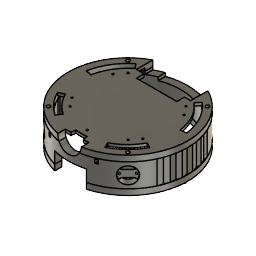
Middle_Layer (Autodesk Fusion 360 design; units mm, degrees)
Autodesk Fusion 360 part; units mm, degrees
note: some values were not read from the file. Set by a fixed rule: which sketch regions a step uses.
sketch "Sketch1" plane through (0, 0, 0) normal (0, 0, 1) x (1, 0, 0)
  circle A0 centre (0, 0) radius 102
  line L0 (0, 0) -> (0, 64) construction
  line L1 (-34.5, 79) -> (34.5, 79)
  line L2 (34.5, 79) -> (34.5, 49)
  line L3 (34.5, 49) -> (-34.5, 49)
  line L4 (-34.5, 49) -> (-34.5, 79)
  line L5 (-34.5, 79) -> (34.5, 49) construction
  line L6 (34.5, 79) -> (-34.5, 49) construction
  point P0 (0, 64)
  dimension "d1" = 204
  dimension "d2" = 64
  dimension "d3" = 69
  dimension "d4" = 30
  constraint coincident A0.centre L0.start
  constraint vertical L0
  constraint horizontal L1
  constraint perpendicular L1 L2
  constraint parallel L1 L3
  constraint parallel L2 L4
  constraint coincident L5 P0
  constraint coincident L6 P0
  constraint coincident P0 L0.end
  measures "d1" diameter of A0
  measures "d2" distance of A0.centre P0
  measures "d3" distance of L2.end L3.end
  measures "d4" distance of L1.end L2.end
extrude "Extrude1" add sketch "Sketch1" along normal blind 5 makes body 1
sketch "Sketch2" plane through (0, 0, 5) normal (0, 0, 1) x (-1, 0, 0)
  line L0 (-34.5, -49) -> (34.5, -49)
  line L1 (34.5, -49) -> (34.5, -79)
  line L2 (34.5, -79) -> (-34.5, -79)
  line L3 (-34.5, -79) -> (-34.5, -49)
  circle A0 centre (0, 0) radius 102
  circle A1 centre (0, 0) radius 70 construction
  line L4 (0, 0) -> (60.6218, 35) construction
  line L5 (0, 0) -> (70, 0) construction
  line L6 (0, 0) -> (60.6218, -35) construction
  line L7 (0, 0) -> (70, 0) construction
  line L8 (0, 0) -> (-60.6218, -35) construction
  line L9 (0, 0) -> (70, 0) construction
  line L10 (0, 0) -> (-60.6218, 35) construction
  line L11 (0, 0) -> (70, 0) construction
  circle A2 centre (60.6218, -35) radius 1.5
  circle A3 centre (60.6218, 35) radius 1.5
  circle A4 centre (-60.6218, -35) radius 1.5
  circle A5 centre (-60.6218, 35) radius 1.5
  dimension "d7" = 140
  dimension "d8" = 30
  dimension "d9" = 30
  dimension "d10" = 150
  dimension "d11" = 150
  dimension "d12" = 3
  dimension "d13" = 3
  dimension "d14" = 3
  dimension "d15" = 3
  constraint concentric A0 A1
  constraint horizontal L5
  constraint coincident A0.centre A1.centre
  constraint horizontal L7
  constraint horizontal L9
  constraint horizontal L11
  constraint coincident L6.end A2.centre
  constraint coincident L4.end A3.centre
  constraint coincident L8.end A4.centre
  constraint coincident L10.end A5.centre
  measures "d7" diameter of A1
  measures "d8" angle of L4 L5
  measures "d9" angle of L6 L7
  measures "d10" angle of L8 L9
  measures "d11" angle of L10 L11
  measures "d12" diameter of A2
  measures "d13" diameter of A3
  measures "d14" diameter of A4
  measures "d15" diameter of A5
extrude "Extrude2" cut sketch "Sketch2" against normal blind 9 contours A2 | A3 | A4 | A5 bodies 1
sketch "Sketch3" plane through (0, 0, 0) normal (0, 0, -1) x (1, 0, 0)
  circle A0 centre (60.6218, 35) radius 1.5
  circle A1 centre (-60.6218, 35) radius 1.5
  circle A2 centre (60.6218, -35) radius 1.5
  circle A3 centre (-60.6218, -35) radius 1.5
  line L0 (-34.5, -49) -> (34.5, -49)
  line L1 (34.5, -49) -> (34.5, -79)
  line L2 (34.5, -79) -> (-34.5, -79)
  line L3 (-34.5, -79) -> (-34.5, -49)
  circle A4 centre (0, 0) radius 102
  circle A5 centre (0, 0) radius 102
  circle A6 centre (0, 0) radius 90
  dimension "d18" = 204
  dimension "d19" = 180
  constraint coincident A4.centre A5.centre
  constraint concentric A5 A6
  measures "d18" diameter of A5
  measures "d19" diameter of A6
extrude "Extrude3" add sketch "Sketch3" along normal blind 5 contours A4 A5 bodies 1
sketch "Sketch4" plane through (0, 0, 0) normal (0, 0, -1) x (1, 0, 0)
  circle A0 centre (0, 0) radius 90
  circle A1 centre (60.6218, 35) radius 1.5
  circle A2 centre (-60.6218, 35) radius 1.5
  circle A3 centre (60.6218, -35) radius 1.5
  circle A4 centre (-60.6218, -35) radius 1.5
  line L0 (-34.5, -49) -> (34.5, -49)
  line L1 (34.5, -49) -> (34.5, -79)
  line L2 (34.5, -79) -> (-34.5, -79)
  line L3 (-34.5, -79) -> (-34.5, -49)
  line L4 (0, 0) -> (0, -49) construction
  line L5 (34.5, -49) -> (-34.5, -49)
  line L6 (-34.5, -49) -> (-34.5, -46.5)
  line L7 (-34.5, -46.5) -> (34.5, -46.5)
  line L8 (34.5, -46.5) -> (34.5, -49)
  dimension "d22" = 2.5
  constraint coincident A0.centre L4.start
  constraint midpoint L0 L4.end
  constraint horizontal L5
  constraint vertical L6
  constraint horizontal L7
  constraint vertical L8
  constraint coincident L0.end L1.start
  measures "d22" distance of L0.end L7.end
extrude "Extrude4" add sketch "Sketch4" along normal blind 54 contours L0 L5 L6 L7 L8 bodies 1
sketch "Sketch5" plane through (0, 0, -5) normal (0, 0, -1) x (1, 0, 0)
  circle A0 centre (0, 0) radius 90
  circle A1 centre (0, 0) radius 102
  circle A2 centre (0, 0) radius 90
  line L0 (0, 0) -> (-88.3346, -51) construction
  line L1 (0, 0) -> (102, 0) construction
  line L2 (0, 0) -> (-88.3346, 51) construction
  line L3 (0, 0) -> (102, 0) construction
  line L4 (0, 0) -> (88.3346, 51) construction
  line L5 (0, 0) -> (102, 0) construction
  line L6 (0, 0) -> (88.3346, -51) construction
  line L7 (0, 0) -> (102, 0) construction
  line L8 (0.3029, -113.7288) -> (0.3029, 125) construction
  line L9 (0, 0) -> (-92.4434, -43.1071) construction
  line L10 (0, 0) -> (102, 0) construction
  line L11 (125, 0) -> (-125, 0) construction
  line L12 (0, 0) -> (-95.8486, -34.8861) construction
  line L13 (0, 0) -> (102, 0) construction
  line L14 (0, 0) -> (-98.5244, -26.3995) construction
  line L15 (0, 0) -> (102, 0) construction
  line L16 (0, 0) -> (-100.4504, -17.7121) construction
  line L17 (0, 0) -> (102, 0) construction
  line L18 (0, 0) -> (-101.6119, -8.8899) construction
  line L19 (0, 0) -> (102, 0) construction
  line L20 (0, 0) -> (-88.3346, 51) construction
  line L21 (0, 0) -> (-92.4434, 43.1071) construction
  line L22 (0, 0) -> (-95.8486, 34.8861) construction
  line L23 (0, 0) -> (-98.5244, 26.3995) construction
  line L24 (0, 0) -> (-100.4504, 17.7121) construction
  line L25 (0, 0) -> (-101.6119, 8.8899) construction
  line L26 (-82.2724, -47.5) -> (-88.3346, -51)
  line L27 (-86.0992, -40.1487) -> (-92.4434, -43.1071)
  line L28 (-82.2724, 47.5) -> (-88.3346, 51)
  line L29 (-86.0992, 40.1487) -> (-92.4434, 43.1071)
  line L30 (-92.4434, -43.1071) -> (-94.909, -34.544)
  line L31 (-94.909, -34.544) -> (-90.6308, -42.2618)
  line L32 (-94.909, -34.544) -> (-96.5926, -25.8819)
  line L33 (-94.909, -34.544) -> (-98.5244, -26.3995)
  line L34 (-96.5926, -25.8819) -> (-99.4656, -17.5385)
  line L35 (-99.4656, -17.5385) -> (-98.5244, -26.3995)
  line L36 (-99.4656, -17.5385) -> (-99.6195, -8.7156)
  line L37 (-99.4656, -17.5385) -> (-101.6119, -8.8899)
  line L38 (-99.6195, -8.7156) -> (-101, 0)
  line L39 (-101, 0) -> (-101.6119, -8.8899)
  line L40 (-101, 0) -> (-99.6195, 8.7156)
  line L41 (-101, 0) -> (-101.6119, 8.8899)
  line L42 (-99.6195, 8.7156) -> (-99.4656, 17.5385)
  line L43 (-99.4656, 17.5385) -> (-101.6119, 8.8899)
  line L44 (-99.4656, 17.5385) -> (-96.5926, 25.8819)
  line L45 (-99.4656, 17.5385) -> (-98.5244, 26.3995)
  line L46 (-96.5926, 25.8819) -> (-94.909, 34.544)
  line L47 (-94.909, 34.544) -> (-98.5244, 26.3995)
  line L48 (-94.909, 34.544) -> (-90.6308, 42.2618)
  line L49 (-94.909, 34.544) -> (-92.4434, 43.1071)
  line L50 (-90.6308, -42.2618) -> (-89.2708, -32.4919)
  line L51 (-89.2708, -32.4919) -> (-96.5926, -25.8819)
  line L52 (-96.5926, -25.8819) -> (-93.5567, -16.4966)
  line L53 (-93.5567, -16.4966) -> (-99.6195, -8.7156)
  line L54 (-99.6195, -8.7156) -> (-95, 0)
  line L55 (-95, 0) -> (-99.6195, 8.7156)
  line L56 (-99.6195, 8.7156) -> (-93.5567, 16.4966)
  line L57 (-93.5567, 16.4966) -> (-96.5926, 25.8819)
  line L58 (-96.5926, 25.8819) -> (-89.2708, 32.4919)
  line L59 (-89.2708, 32.4919) -> (-90.6308, 42.2618)
  line L60 (-91.763, -24.5878) -> (-91.763, 24.5878)
  arc A3 (-82.2724, 47.5) -> (-91.763, 24.5878) centre (0, 0) ccw
  arc A4 (-91.763, -24.5878) -> (-82.2724, -47.5) centre (0, 0) ccw
  line L61 (0.6059, 0) -> (88.9405, -51) construction
  line L62 (0.6059, 0) -> (93.0493, -43.1071) construction
  line L63 (0.6059, 0) -> (96.4545, -34.8861) construction
  line L64 (0.6059, 0) -> (99.1303, -26.3995) construction
  line L65 (0.6059, 0) -> (101.0563, -17.7121) construction
  line L66 (0.6059, 0) -> (102.2178, -8.8899) construction
  line L67 (-124.3941, 0) -> (125.6059, 0) construction
  line L68 (0.6059, 0) -> (102.2178, 8.8899) construction
  line L69 (0.6059, 0) -> (101.0563, 17.7121) construction
  line L70 (0.6059, 0) -> (99.1303, 26.3995) construction
  line L71 (0.6059, 0) -> (96.4545, 34.8861) construction
  line L72 (0.6059, 0) -> (93.0493, 43.1071) construction
  line L73 (0.6059, 0) -> (88.9405, 51) construction
  line L74 (92.5513, -42.8749) -> (86.2071, -39.9165)
  line L75 (88.3346, -51) -> (82.2724, -47.5)
  line L76 (88.3346, 51) -> (82.2724, 47.5)
  line L77 (92.5513, 42.8749) -> (86.2071, 39.9165)
  line L78 (92.5513, -42.8749) -> (94.9796, -34.3492)
  line L79 (94.9796, -34.3492) -> (90.7179, -42.0199)
  line L80 (94.9796, -34.3492) -> (98.5649, -26.248)
  line L81 (94.9796, -34.3492) -> (96.6331, -25.7304)
  line L82 (98.5649, -26.248) -> (99.4838, -17.4348)
  line L83 (99.4838, -17.4348) -> (96.6331, -25.7304)
  line L84 (99.4838, -17.4348) -> (101.6164, -8.8373)
  line L85 (99.4838, -17.4348) -> (99.6241, -8.663)
  line L86 (101.6164, -8.8373) -> (101, 0)
  line L87 (101, 0) -> (99.6241, -8.663)
  line L88 (101, 0) -> (101.6164, 8.8373)
  line L89 (101, 0) -> (99.6241, 8.663)
  line L90 (101.6164, 8.8373) -> (99.4838, 17.4348)
  line L91 (99.4838, 17.4348) -> (99.6241, 8.663)
  line L92 (99.4838, 17.4348) -> (98.5649, 26.248)
  line L93 (99.4838, 17.4348) -> (96.6331, 25.7304)
  line L94 (98.5649, 26.248) -> (94.9796, 34.3492)
  line L95 (96.6331, 25.7304) -> (94.9796, 34.3492)
  line L96 (94.9796, 34.3492) -> (92.5513, 42.8749)
  line L97 (94.9796, 34.3492) -> (90.7387, 42.0296)
  line L98 (90.7387, 42.0296) -> (89.3415, 32.2971)
  line L99 (89.3415, 32.2971) -> (96.6331, 25.7304)
  line L100 (96.6331, 25.7304) -> (93.5749, 16.393)
  line L101 (93.5749, 16.393) -> (99.6241, 8.663)
  line L102 (99.6241, 8.663) -> (95, 0)
  line L103 (95, 0) -> (99.6241, -8.663)
  line L104 (99.6241, -8.663) -> (93.5749, -16.393)
  line L105 (93.5749, -16.393) -> (96.6331, -25.7304)
  line L106 (96.6331, -25.7304) -> (89.3415, -32.2971)
  line L107 (89.3415, -32.2971) -> (90.7179, -42.0199)
  line L108 (89.3415, -32.2971) -> (93.5749, 16.393)
  arc A5 (86.7536, 49.7374) -> (86.6025, 50) centre (0, 0) ccw
  arc A6 (87.4686, -50.5) -> (87.6196, -50.2374) centre (0, 0) ccw
  arc A7 (87.6196, 50.2374) -> (87.4686, 50.5) centre (0, 0) ccw
  arc A8 (-92.4434, -43.1071) -> (92.5513, -42.8749) centre (0, 0) ccw
  arc A9 (92.5513, 42.8749) -> (-92.4434, 43.1071) centre (0, 0) ccw
  arc A10 (82.2724, -47.5) -> (89.3415, -32.2971) centre (0, 0) ccw
  arc A11 (93.5749, 16.393) -> (82.2724, 47.5) centre (0, 0) ccw
  arc A12 (86.6025, -50) -> (86.7536, -49.7374) centre (0, 0) ccw
  arc A13 (90.7387, -42.0296) -> (90.8667, -41.7522) centre (0, 0) ccw
  line L109 (82.2724, -47.5) -> (77.9423, -45)
  line L110 (86.2071, -39.9165) -> (81.6756, -37.8034)
  line L111 (86.2071, 39.9165) -> (81.6756, 37.8034)
  line L112 (82.2724, 47.5) -> (77.9423, 45)
  line L113 (-77.9423, -45) -> (-82.2724, -47.5)
  line L114 (-81.5677, -38.0356) -> (-86.0992, -40.1487)
  line L115 (-77.9423, 45) -> (-82.2724, 47.5)
  line L116 (-81.5677, 38.0356) -> (-86.0992, 40.1487)
  dimension "d25" = 204
  dimension "d26" = 180
  dimension "d27" = 150
  dimension "d28" = 150
  dimension "d29" = 30
  dimension "d30" = 30
  dimension "d31" = 155
  dimension "d32" = 160
  dimension "d33" = 165
  dimension "d34" = 170
  dimension "d35" = 175
  dimension "d36" = 190
  dimension "d37" = 202
  dimension "d38" = 200
  constraint coincident A0.centre A1.centre
  constraint horizontal L1
  constraint horizontal L3
  constraint horizontal L5
  constraint horizontal L7
  constraint vertical L8
  constraint horizontal L10
  constraint horizontal L11
  constraint horizontal L13
  constraint horizontal L15
  constraint horizontal L17
  constraint horizontal L19
  constraint symmetric A0.centre L11 A1.centre
  constraint symmetric L0.end L11 L2.end
  constraint symmetric L9.end L11 L21.end
  constraint symmetric L11 L12.end L22.end
  constraint symmetric L11 L14.end L23.end
  constraint symmetric L11 A0.centre A1.centre
  constraint symmetric L11 L16.end L24.end
  constraint symmetric L11 L18.end L25.end
  constraint coincident L0 L26.start
  constraint coincident L27.start A4
  constraint coincident L9 L27.start
  constraint coincident L20 L28.start
  constraint coincident L21 L29.start
  constraint coincident L29.start A3
  constraint coincident L12 L30.end
  constraint coincident L27 L31.end
  constraint coincident L14 L32.end
  constraint coincident L16 L34.end
  constraint coincident L18 L36.end
  constraint coincident L11 L38.end
  constraint coincident L25 L40.end
  constraint coincident L24 L42.end
  constraint coincident L23 L44.end
  constraint coincident L22 L46.end
  constraint coincident L29 L48.end
  constraint coincident L12 L50.end
  constraint coincident L50.end A4
  constraint coincident L16 L52.end
  constraint coincident L11 L54.end
  constraint coincident L24 L56.end
  constraint coincident L58.end A3
  constraint coincident L22 L58.end
  constraint coincident L14 L60.start
  constraint coincident L23 L60.end
  constraint concentric A3 A11
  constraint coincident L6 L75.end
  constraint coincident L6 A12.start
  constraint coincident L6 A6.start
  constraint coincident L4 L76.end
  constraint coincident L4 A5.end
  constraint coincident L4 A7.end
  constraint concentric A3 A4
  constraint symmetric A0.centre L8 L61.start
  constraint symmetric L0.end L8 L61.end
  constraint symmetric L2.end L8 L73.end
  constraint symmetric L8 A0.centre L61.start
  constraint symmetric L8 L9.end L62.end
  constraint symmetric L8 L11.start L67.start
  constraint symmetric L8 L11.end L67.end
  constraint symmetric L8 L12.end L63.end
  constraint symmetric L8 L14.end L64.end
  constraint symmetric L8 L16.end L65.end
  constraint symmetric L8 L18.end L66.end
  constraint symmetric L8 L21.end L72.end
  constraint symmetric L8 L22.end L71.end
  constraint symmetric L8 L23.end L70.end
  constraint symmetric L8 L24.end L69.end
  constraint symmetric L8 L25.end L68.end
  constraint coincident L62 L74.start
  constraint coincident L62 L74.end
  constraint coincident L74.end A10
  constraint coincident L72 L77.start
  constraint coincident L77.end A11
  constraint coincident L72 L77.end
  constraint coincident L63 L78.end
  constraint coincident L62 L79.end
  constraint coincident L64 L80.end
  constraint coincident A1 L80.end
  constraint coincident L64 L81.end
  constraint coincident L65 L82.end
  constraint coincident L66 L84.end
  constraint coincident L66 L85.end
  constraint coincident L68 L88.end
  constraint coincident L68 L89.end
  constraint coincident L69 L90.end
  constraint coincident L70 L92.end
  constraint coincident L70 L93.end
  constraint coincident L71 L94.end
  constraint coincident L77 L97.end
  constraint coincident L98.end A11
  constraint coincident L71 L98.end
  constraint coincident L69 L100.end
  constraint coincident L65 L104.end
  constraint coincident L63 L106.end
  constraint coincident L73 A5.start
  constraint concentric A5 A13
  constraint coincident L73 A7.start
  constraint concentric A6 A7
  constraint concentric A8 A9
  constraint concentric A10 A11
  constraint coincident L79 A13.end
  constraint coincident L61 A6.end
  constraint coincident L61 A12.end
  constraint coincident L62 A13.start
  constraint concentric A12 A13
  constraint coincident A2 L109.end
  constraint coincident L6 L109.end
  constraint coincident L62 L110.end
  constraint coincident A2 L110.end
  constraint coincident L72 L111.end
  constraint coincident A2 L111.end
  constraint coincident A2 L112.end
  constraint coincident L4 L112.end
  constraint coincident L0 L113.start
  constraint coincident A2 L113.start
  constraint coincident L9 L114.start
  constraint coincident A2 L114.start
  constraint coincident L2 L115.start
  constraint coincident A2 L115.start
  constraint parallel L28 L115
  constraint coincident A2 L116.start
  constraint coincident L21 L116.start
  measures "d25" diameter of A8
  measures "d26" diameter of A2
  measures "d27" angle of L0 L1
  measures "d28" angle of L2 L3
  measures "d29" angle of L4 L5
  measures "d30" angle of L6 L7
  measures "d31" angle of L9 L10
  measures "d32" angle of L12 L13
  measures "d33" angle of L14 L15
  measures "d34" angle of L16 L17
  measures "d35" angle of L18 L19
  measures "d36" diameter of A10
  measures "d37" diameter of A6
  measures "d38" diameter of A12
extrude "Extrude5" add sketch "Sketch5" along normal blind 40 separate body contours A0 A2 A11 L111 L112 | A0 A2 A10 L109 L110 | A0 A1 A2 L28 L76 A9 L112 L115 | A1 L76 L77 A9 A11 | L77 L98 A11 | A0 A1 A2 L26 L75 A8 L109 L113 | L74 L107 A10 | A1 L74 L75 A8 A10 | A0 A2 A3 L115 L116 | L77 L96 L97 | L99 L100 A11 | A0 A2 A4 L113 L114 | L101 L102 L103 L104 L105 L106 L108 | A1 L28 L29 A3 A9 | L92 L93 L94 L95 | A1 L26 L27 A4 A8 | L74 L78 L79 A13 | L80 L81 L82 L83 | L29 L59 A3 | L88 L89 L90 L91 | L27 L50 A4 | L84 L85 L86 L87 | L29 L48 L49 | L51 L52 L53 L54 L55 L56 L57 L58 L60 A3 A4 | L27 L30 L31 | L44 L45 L46 L47 | L32 L33 L34 L35 | L40 L41 L42 L43 | L36 L37 L38 L39 makes body 2 at (-87.956, 51.6502, -18.3333)
sketch "Sketch6" plane through (0, 0, -45) normal (0, 0, -1) x (1, 0, 0)
  line L0 (86.2071, -39.9165) -> (81.6756, -37.8034)
  arc A0 (-81.5677, -38.0356) -> (81.6756, -37.8034) centre (0, 0) ccw
  line L1 (-81.5677, -38.0356) -> (-86.0992, -40.1487)
  arc A1 (-89.2708, -32.4919) -> (-86.0992, -40.1487) centre (0, 0) ccw
  line L2 (-89.2708, -32.4919) -> (-90.6308, -42.2618)
  line L3 (-90.6308, -42.2618) -> (-94.909, -34.544)
  line L4 (-94.909, -34.544) -> (-92.4434, -43.1071)
  arc A2 (-92.4434, -43.1071) -> (92.5513, -42.8749) centre (0, 0) ccw
  line L5 (92.5513, -42.8749) -> (94.9796, -34.3492)
  line L6 (94.9796, -34.3492) -> (90.8667, -41.7522)
  arc A3 (90.7387, -42.0296) -> (90.8667, -41.7522) centre (0, 0) ccw
  line L7 (90.7387, -42.0296) -> (90.7179, -42.0199)
  line L8 (90.7179, -42.0199) -> (89.3415, -32.2971)
  arc A4 (86.2071, -39.9165) -> (89.3415, -32.2971) centre (0, 0) ccw
  circle A5 centre (0, 0) radius 102
  circle A6 centre (0, 0) radius 90
  dimension "d41" = 204
  dimension "d42" = 180
  constraint concentric A3 A5
  constraint concentric A5 A6
  measures "d41" diameter of A5
  measures "d42" diameter of A6
extrude "Extrude6" add sketch "Sketch6" along normal blind 10 separate body contours L0 A0 L1 A1 L2 L3 L4 A2 L5 L6 A3 L7 L8 A4 A5 A6 | L0 L1 A1 L2 L3 L4 L5 L6 A3 L7 L8 A4 A5 A6 makes body 3
sketch "Sketch7" plane through (0, 0, -55) normal (0, 0, -1) x (1, 0, 0)
  circle A0 centre (0, 0) radius 90
  circle A1 centre (0, 0) radius 102
  circle A2 centre (0, 0) radius 96 construction
  circle A3 centre (96, 0) radius 2.975
  circle A4 centre (-96, 0) radius 2.975
  dimension "d45" = 192
  dimension "d46" = 5.95
  dimension "d47" = 5.95
  constraint coincident A0.centre A1.centre
  constraint coincident A2 A3.centre
  constraint coincident A2 A4.centre
  measures "d45" diameter of A2
  measures "d46" diameter of A3
  measures "d47" diameter of A4
extrude "Extrude7" add sketch "Sketch7" along normal blind 3.95 contours A3 | A4 bodies 3
sketch "Sketch8" plane through (0, 0, 0) normal (0, 0, -1) x (1, 0, 0)
  line L0 (-34.5, -49) -> (-34.5, -46.5)
  line L1 (-34.5, -46.5) -> (34.5, -46.5)
  line L2 (34.5, -46.5) -> (34.5, -49)
  line L3 (34.5, -49) -> (34.5, -79)
  line L4 (34.5, -79) -> (-34.5, -79)
  line L5 (-34.5, -79) -> (-34.5, -49)
  circle A0 centre (-60.6218, -35) radius 1.5
  circle A1 centre (60.6218, -35) radius 1.5
  circle A2 centre (-60.6218, 35) radius 1.5
  circle A3 centre (60.6218, 35) radius 1.5
  circle A4 centre (0, 0) radius 90
  circle A5 centre (0, 0) radius 70 construction
  line L6 (0, 0) -> (0, 70) construction
  line L7 (0, 0) -> (49.4975, 49.4975) construction
  line L8 (0, 0) -> (49.4975, -49.4975) construction
  line L9 (0, 0) -> (70, 0) construction
  line L10 (0, 0) -> (-49.4975, -49.4975) construction
  line L11 (0, 0) -> (70, 0) construction
  line L12 (0, 0) -> (-49.4975, 49.4975) construction
  line L13 (0, 0) -> (70, 0) construction
  circle A6 centre (0, 70) radius 1.5
  circle A7 centre (49.4975, 49.4975) radius 1.5
  circle A8 centre (-49.4975, 49.4975) radius 1.5
  circle A9 centre (49.4975, -49.4975) radius 1.5
  circle A10 centre (-49.4975, -49.4975) radius 1.5
  dimension "d50" = 140
  dimension "d51" = 135
  dimension "d52" = 45
  dimension "d53" = 135
  dimension "d54" = 135
  dimension "d55" = 3
  dimension "d56" = 3
  dimension "d57" = 3
  dimension "d58" = 3
  dimension "d59" = 3
  constraint concentric A4 A5
  constraint coincident A4.centre A5.centre
  constraint coincident A5 L6.end
  constraint vertical L6
  constraint horizontal L9
  constraint horizontal L11
  constraint horizontal L13
  constraint coincident L6.end A6.centre
  constraint coincident L7.end A7.centre
  constraint coincident L12.end A8.centre
  constraint coincident L8.end A9.centre
  constraint coincident L10.end A10.centre
  measures "d50" diameter of A5
  measures "d51" angle of L6 L7
  measures "d52" angle of L8 L9
  measures "d53" angle of L10 L11
  measures "d54" angle of L12 L13
  measures "d55" diameter of A6
  measures "d56" diameter of A7
  measures "d57" diameter of A8
  measures "d58" diameter of A9
  measures "d59" diameter of A10
extrude "Extrude8" cut sketch "Sketch8" against normal blind 8 contours A6 | A7 | A8 | A9 | A10 bodies 1
sketch "Sketch9" plane through (0, 0, 0) normal (0, 0, -1) x (1, 0, 0)
  circle A0 centre (49.4975, 49.4975) radius 1.5
  circle A1 centre (-49.4975, -49.4975) radius 1.5
  circle A2 centre (-49.4975, 49.4975) radius 1.5
  circle A3 centre (49.4975, -49.4975) radius 1.5
  circle A4 centre (0, 70) radius 1.5
  line L0 (-34.5, -49) -> (-34.5, -46.5)
  line L1 (-34.5, -46.5) -> (34.5, -46.5)
  line L2 (34.5, -46.5) -> (34.5, -49)
  line L3 (34.5, -49) -> (34.5, -79)
  line L4 (34.5, -79) -> (-34.5, -79)
  line L5 (-34.5, -79) -> (-34.5, -49)
  circle A5 centre (-60.6218, -35) radius 1.5
  circle A6 centre (60.6218, -35) radius 1.5
  circle A7 centre (-60.6218, 35) radius 1.5
  circle A8 centre (60.6218, 35) radius 1.5
  circle A9 centre (0, 0) radius 90
  line L6 (0, 0) -> (0, 55) construction
  line L7 (40.5, 38.5) -> (-40.5, 38.5) construction
  line L8 (-40.5, 38.5) -> (-40.5, 71.5) construction
  line L9 (-40.5, 71.5) -> (40.5, 71.5) construction
  line L10 (40.5, 71.5) -> (40.5, 38.5) construction
  line L11 (40.5, 38.5) -> (-40.5, 71.5) construction
  line L12 (-40.5, 38.5) -> (40.5, 71.5) construction
  circle A10 centre (-40.5, 71.5) radius 2.9
  line L13 (-40.5, 71.5) -> (16.5, 71.5) construction
  line L14 (16.5, 71.5) -> (16.5, 41.5) construction
  circle A11 centre (16.5, 41.5) radius 2.9
  point P0 (0, 55)
  dimension "d62" = 55
  dimension "d63" = 81
  dimension "d64" = 33
  dimension "d65" = 5.8
  dimension "d66" = 57
  dimension "d67" = 30
  dimension "d68" = 5.8
  constraint coincident A9.centre L6.start
  constraint perpendicular L4 L6
  constraint horizontal L7
  constraint perpendicular L7 L8
  constraint parallel L7 L9
  constraint parallel L8 L10
  constraint coincident L11 P0
  constraint coincident L12 P0
  constraint coincident P0 L6.end
  constraint coincident L8.end L9.start
  constraint parallel L9 L13
  constraint perpendicular L13 L14
  constraint coincident L14.end A11.centre
  measures "d62" distance of A9.centre P0
  measures "d63" distance of L8.end L9.end
  measures "d64" distance of L7.end L8.end
  measures "d65" diameter of A10
  measures "d66" distance of L8.end L13.end
  measures "d67" distance of L13.end L14.end
  measures "d68" diameter of A11
extrude "Extrude9" add sketch "Sketch9" along normal blind 5 contours A10 | A11 bodies 1
ref_plane "WorkPlane1" through (0, -102, -16.1846) normal (0, -1, 0) x (1, 0, 0)
sketch "Sketch10" plane through (0, -102, 0) normal (0, -1, 0) x (-1, 0, 0)
  line L0 (0, 55) -> (0, 40) construction
  line L1 (-27, 55) -> (27, 55)
  line L2 (27, 55) -> (27, 25)
  line L3 (27, 25) -> (-27, 25)
  line L4 (-27, 25) -> (-27, 55)
  line L5 (-27, 55) -> (27, 25) construction
  line L6 (27, 55) -> (-27, 25) construction
  line L7 (0, 55) -> (0, 10) construction
  line L8 (0, 10) -> (-40, 10) construction
  line L9 (0, 10) -> (40, 10) construction
  line L10 (-42, 13) -> (-38, 13)
  line L11 (-38, 13) -> (-38, 7)
  line L12 (-38, 7) -> (-42, 7)
  line L13 (-42, 7) -> (-42, 13)
  line L14 (-42, 13) -> (-38, 7) construction
  line L15 (-38, 13) -> (-42, 7) construction
  line L16 (38, 13) -> (42, 13)
  line L17 (42, 13) -> (42, 7)
  line L18 (42, 7) -> (38, 7)
  line L19 (38, 7) -> (38, 13)
  line L20 (38, 13) -> (42, 7) construction
  line L21 (42, 13) -> (38, 7) construction
  point P0 (0, 40)
  point P1 (-40, 10)
  point P2 (40, 10)
  dimension "d72" = 15
  dimension "d73" = 54
  dimension "d74" = 30
  dimension "d75" = 40
  dimension "d76" = 40
  dimension "d77" = 4
  dimension "d78" = 6
  dimension "d79" = 4
  dimension "d80" = 6
  constraint vertical L0
  constraint horizontal L1
  constraint perpendicular L1 L2
  constraint parallel L1 L3
  constraint parallel L2 L4
  constraint coincident L5 P0
  constraint coincident L6 P0
  constraint coincident P0 L0.end
  constraint perpendicular L3 L7
  constraint perpendicular L7 L8
  constraint perpendicular L7 L9
  constraint horizontal L10
  constraint perpendicular L10 L11
  constraint parallel L10 L12
  constraint parallel L11 L13
  constraint coincident L14 P1
  constraint coincident L15 P1
  constraint coincident P1 L8.end
  constraint horizontal L16
  constraint perpendicular L16 L17
  constraint parallel L16 L18
  constraint parallel L17 L19
  constraint coincident L20 P2
  constraint coincident L21 P2
  constraint coincident P2 L9.end
  measures "d72" distance of L0.start P0
  measures "d73" distance of L2.end L3.end
  measures "d74" distance of L1.end L2.end
  measures "d75" distance of L7.end P1
  measures "d76" distance of L7.end P2
  measures "d77" distance of L11.end L12.end
  measures "d78" distance of L10.end L11.end
  measures "d79" distance of L17.end L18.end
  measures "d80" distance of L16.end L17.end
extrude "Extrude10" cut sketch "Sketch10" against normal blind 25 bodies 2 3
ref_plane "WorkPlane2" through (0, 102, -29.3168) normal (0, 1, 0) x (-1, 0, 0)
sketch "Sketch11" plane through (0, 102, 0) normal (0, 1, 0) x (1, 0, 0)
  line L0 (0, 55) -> (0, -2) construction
  line L1 (-32.5, 15) -> (32.5, 15)
  line L2 (32.5, 15) -> (32.5, -19)
  line L3 (32.5, -19) -> (-32.5, -19)
  line L4 (-32.5, -19) -> (-32.5, 15)
  line L5 (-32.5, 15) -> (32.5, -19) construction
  line L6 (32.5, 15) -> (-32.5, -19) construction
  line L7 (0, 55) -> (0, 10)
  line L8 (0, 10) -> (32.5, 10)
  line L9 (32.5, 10) -> (45, 10)
  line L10 (45, 10) -> (45, -5)
  line L11 (45, -5) -> (32.5, -5)
  line L12 (32.5, -5) -> (32.5, 10)
  point P0 (0, -2)
  dimension "d84" = 57
  dimension "d85" = 65
  dimension "d86" = 34
  dimension "d87" = 45
  constraint vertical L0
  constraint horizontal L1
  constraint perpendicular L1 L2
  constraint parallel L1 L3
  constraint parallel L2 L4
  constraint coincident L5 P0
  constraint coincident L6 P0
  constraint coincident P0 L0.end
  constraint parallel L0 L7
  constraint coincident L2 L8.end
  constraint perpendicular L2 L8
  constraint horizontal L9
  constraint vertical L10
  constraint horizontal L11
  constraint vertical L12
  measures "d84" distance of L0.start P0
  measures "d85" distance of L2.end L3.end
  measures "d86" distance of L1.end L2.end
  measures "d87" distance of L0.start L7.end
extrude "Extrude11" cut sketch "Sketch11" against normal blind 40 bodies 1 2
ref_plane "WorkPlane3" through (-72.1249, -72.1249, -19.7035) normal (-0.707107, -0.707107, 0) x (0.707107, -0.707107, 0)
sketch "Sketch12" plane through (-72.1249, -72.1249, 0) normal (-0.707107, -0.707107, 0) x (0.707107, -0.707107, 0)
  circle A0 centre (0.3377, -27) radius 14
  line L0 (8.3377, -33) -> (-7.6623, -33)
  line L1 (-7.6623, -33) -> (-7.6623, -21)
  line L2 (-7.6623, -21) -> (8.3377, -21)
  line L3 (8.3377, -21) -> (8.3377, -33)
  line L4 (8.3377, -33) -> (-7.6623, -21) construction
  line L5 (-7.6623, -33) -> (8.3377, -21) construction
  line L6 (0.3377, -27) -> (11.5377, -35.4)
  line L7 (0.3377, -27) -> (11.5377, -18.6)
  line L8 (0.3377, -27) -> (-10.8623, -18.6)
  line L9 (0.3377, -27) -> (-10.7934, -35.4911)
  line L10 (0.3377, -27) -> (10.8377, -27) construction
  line L11 (0.3377, -27) -> (-10.1623, -27) construction
  circle A1 centre (10.8377, -27) radius 1.625
  circle A2 centre (-10.1623, -27) radius 1.625
  point P0 (0.3377, -27)
  dimension "d91" = 28
  dimension "d92" = 16
  dimension "d93" = 12
  dimension "d94" = 10.5
  dimension "d95" = 10.5
  dimension "d96" = 3.25
  dimension "d97" = 3.25
  constraint horizontal L0
  constraint perpendicular L0 L1
  constraint parallel L0 L2
  constraint parallel L1 L3
  constraint coincident L4 P0
  constraint coincident L5 P0
  constraint coincident P0 A0.centre
  constraint coincident A0 L6.end
  constraint parallel L4 L6
  constraint coincident A0 L7.end
  constraint coincident A0 L8.end
  constraint parallel L4 L8
  constraint coincident A0 L9.end
  constraint perpendicular L3 L10
  constraint perpendicular L1 L11
  constraint coincident L10.end A1.centre
  constraint coincident L11.end A2.centre
  measures "d91" diameter of A0
  measures "d92" distance of L1.end L2.end
  measures "d93" distance of L0.end L1.end
  measures "d94" distance of P0 L10.end
  measures "d95" distance of P0 L11.end
  measures "d96" diameter of A1
  measures "d97" diameter of A2
extrude "Extrude12" cut sketch "Sketch12" against normal blind 25 contours A0 L2 L7 L8 | A0 L0 L6 L9 | A1 | A2 bodies 2
extrude "Extrude13" cut sketch "Sketch12" against normal blind 4 contours A0 L3 L6 L7 | A0 L0 L1 L8 L9 | L2 L7 L8 | L3 L6 L7 | L0 L6 L9 | L0 L1 L8 L9 bodies 2
sketch "Sketch13" plane through (0, -102, 0) normal (0, -1, 0) x (-1, 0, 0)
  circle A0 centre (0, -5) radius 20
  dimension "d102" = 40
  measures "d102" diameter of A0
extrude "Extrude14" cut sketch "Sketch13" against normal blind 15 bodies 1 2
ref_plane "WorkPlane4" through (72.1249, -72.1249, -16.7961) normal (0.707107, -0.707107, 0) x (0.707107, 0.707107, 0)
sketch "Sketch14" plane through (72.1249, -72.1249, 0) normal (0.707107, -0.707107, 0) x (0.707107, 0.707107, 0)
  circle A0 centre (0, -25) radius 14
  line L0 (8, -19) -> (-8, -19)
  line L1 (-8, -19) -> (-8, -31)
  line L2 (-8, -31) -> (8, -31)
  line L3 (8, -31) -> (8, -19)
  line L4 (8, -19) -> (-8, -31) construction
  line L5 (-8, -19) -> (8, -31) construction
  line L6 (0, -25) -> (-10.9974, -33.6636)
  line L7 (0, -25) -> (11.2, -16.6)
  line L8 (0, -25) -> (11.2, -33.4)
  line L9 (0, -25) -> (-12.6598, -15.5052)
  line L10 (0, -25) -> (-10.5, -25) construction
  line L11 (0, -25) -> (10.5, -25) construction
  circle A1 centre (-10.5, -25) radius 1.625
  circle A2 centre (10.5, -25) radius 1.625
  point P0 (0, -25)
  dimension "d106" = 28
  dimension "d107" = 16
  dimension "d108" = 12
  dimension "d109" = 10.5
  dimension "d110" = 10.5
  dimension "d111" = 3.25
  dimension "d112" = 3.25
  constraint horizontal L0
  constraint perpendicular L0 L1
  constraint parallel L0 L2
  constraint parallel L1 L3
  constraint coincident L4 P0
  constraint coincident L5 P0
  constraint coincident P0 A0.centre
  constraint coincident A0 L6.end
  constraint coincident A0 L7.end
  constraint parallel L4 L7
  constraint coincident A0 L8.end
  constraint parallel L5 L8
  constraint parallel L5 L9
  constraint perpendicular L1 L10
  constraint perpendicular L3 L11
  constraint coincident L10.end A1.centre
  constraint coincident L11.end A2.centre
  measures "d106" diameter of A0
  measures "d107" distance of L1.end L2.end
  measures "d108" distance of L0.end L1.end
  measures "d109" distance of P0 L10.end
  measures "d110" distance of P0 L11.end
  measures "d111" diameter of A1
  measures "d112" diameter of A2
extrude "Extrude15" cut sketch "Sketch14" against normal blind 40 contours A0 L0 L7 L9 | A0 L2 L6 L8 | A1 | A2 bodies 2
extrude "Extrude16" cut sketch "Sketch14" against normal blind 4 contours A0 L3 L7 L8 | A0 L1 L2 L6 L9 | L0 L7 L9 | L3 L7 L8 | L2 L6 L8 | L1 L2 L6 L9 bodies 2
sketch "Sketch15" plane through (0, 0, -55) normal (0, 0, -1) x (1, 0, 0)
  line L0 (-27, 85.8545) -> (-27, 98.3616)
  arc A0 (-27, 98.3616) -> (27, 98.3616) centre (0, 0) ccw
  line L1 (27, 98.3616) -> (27, 85.8545)
  arc A1 (-27, 85.8545) -> (27, 85.8545) centre (0, 0) ccw
  circle A2 centre (96, 0) radius 2.975
  circle A3 centre (-96, 0) radius 2.975
  circle A4 centre (0, 0) radius 96 construction
  circle A5 centre (0, -96) radius 2.95
  dimension "d117" = 192
  dimension "d118" = 5.9
  constraint concentric A0 A4
  constraint coincident A4 A5.centre
  measures "d117" diameter of A4
  measures "d118" diameter of A5
extrude "Extrude17" add sketch "Sketch15" along normal blind 3.9 contours A5 bodies 3
sketch "Sketch16" plane through (0, 0, 5) normal (0, 0, 1) x (-1, 0, 0)
  circle A0 centre (60.6218, -35) radius 1.5
  circle A1 centre (-60.6218, -35) radius 1.5
  circle A2 centre (60.6218, 35) radius 1.5
  circle A3 centre (-60.6218, 35) radius 1.5
  circle A4 centre (0, 70) radius 1.5
  circle A5 centre (-49.4975, -49.4975) radius 1.5
  circle A6 centre (49.4975, 49.4975) radius 1.5
  circle A7 centre (49.4975, -49.4975) radius 1.5
  circle A8 centre (-49.4975, 49.4975) radius 1.5
  line L0 (20, 100.02) -> (20, 87)
  line L1 (20, 87) -> (-20, 87)
  line L2 (-20, 87) -> (-20, 100.02)
  arc A9 (-20, 100.02) -> (-45, -91.5369) centre (0, 0) ccw
  line L3 (-45, -91.5369) -> (-45, -62)
  line L4 (-45, -62) -> (-34.5, -62)
  line L5 (-34.5, -62) -> (-34.5, -49)
  line L6 (-34.5, -49) -> (34.5, -49)
  line L7 (34.5, -49) -> (34.5, -79)
  line L8 (34.5, -79) -> (32.5, -79)
  line L9 (32.5, -79) -> (32.5, -96.6838)
  arc A10 (32.5, -96.6838) -> (20, 100.02) centre (0, 0) ccw
  circle A11 centre (0, 0) radius 96 construction
  line L10 (0, 0) -> (-67.8823, -67.8823) construction
  line L11 (0, 0) -> (96, 0) construction
  line L12 (0, 0) -> (-67.8823, 67.8823) construction
  line L13 (0, 0) -> (96, 0) construction
  line L14 (0, 0) -> (67.8823, -67.8823) construction
  line L15 (0, 0) -> (96, 0) construction
  line L16 (0, 0) -> (67.8823, 67.8823) construction
  line L17 (0, 0) -> (96, 0) construction
  circle A12 centre (-67.8823, -67.8823) radius 3
  circle A13 centre (67.8823, -67.8823) radius 3
  circle A14 centre (67.8823, 67.8823) radius 3
  circle A15 centre (-67.8823, 67.8823) radius 3
  dimension "d121" = 192
  dimension "d122" = 135
  dimension "d123" = 135
  dimension "d124" = 45
  dimension "d125" = 45
  dimension "d126" = 6
  dimension "d127" = 6
  dimension "d128" = 6
  dimension "d129" = 6
  constraint coincident A9.centre A10.centre
  constraint horizontal L11
  constraint horizontal L13
  constraint horizontal L15
  constraint horizontal L17
  constraint coincident L10.end A12.centre
  constraint coincident L14.end A13.centre
  constraint coincident L16.end A14.centre
  constraint coincident L12.end A15.centre
  measures "d121" diameter of A11
  measures "d122" angle of L10 L11
  measures "d123" angle of L12 L13
  measures "d124" angle of L14 L15
  measures "d125" angle of L16 L17
  measures "d126" diameter of A12
  measures "d127" diameter of A13
  measures "d128" diameter of A14
  measures "d129" diameter of A15
extrude "Extrude18" cut sketch "Sketch16" against normal blind 5 contours A12 | A13 | A14 | A15 bodies 1
sketch "Sketch17" plane through (0, 0, 0) normal (0, 0, -1) x (1, 0, 0)
  line L0 (-19.3649, 87) -> (-19.3649, 87.892)
  arc A0 (-19.3649, 87.892) -> (-32.5, -83.9271) centre (0, 0) ccw
  line L1 (-32.5, -83.9271) -> (-32.5, -79)
  line L2 (-32.5, -79) -> (-34.5, -79)
  line L3 (-34.5, -79) -> (-34.5, -49)
  line L4 (-34.5, -49) -> (-34.5, -46.5)
  line L5 (-34.5, -46.5) -> (34.5, -46.5)
  line L6 (34.5, -46.5) -> (34.5, -49)
  line L7 (34.5, -49) -> (34.5, -62)
  line L8 (34.5, -62) -> (45, -62)
  line L9 (45, -62) -> (45, -77.9423)
  arc A1 (45, -77.9423) -> (19.3649, 87.892) centre (0, 0) ccw
  line L10 (19.3649, 87.892) -> (19.3649, 87)
  line L11 (19.3649, 87) -> (-19.3649, 87)
  circle A2 centre (-40.5, 71.5) radius 2.9
  circle A3 centre (16.5, 41.5) radius 2.9
  circle A4 centre (49.4975, 49.4975) radius 1.5
  circle A5 centre (-49.4975, -49.4975) radius 1.5
  circle A6 centre (-49.4975, 49.4975) radius 1.5
  circle A7 centre (49.4975, -49.4975) radius 1.5
  circle A8 centre (0, 70) radius 1.5
  circle A9 centre (-60.6218, -35) radius 1.5
  circle A10 centre (60.6218, -35) radius 1.5
  circle A11 centre (-60.6218, 35) radius 1.5
  circle A12 centre (60.6218, 35) radius 1.5
  circle A13 centre (0, 0) radius 90
  circle A14 centre (0, 0) radius 80
  line L12 (0, 0) -> (57.2638, -69.4324)
  line L13 (0, 0) -> (89.3486, -10.8083)
  line L14 (0, 0) -> (79.3816, 42.4094)
  line L15 (0, 0) -> (40.9728, 80.1326)
  line L16 (0, 0) -> (-56.4415, -70.1025)
  line L17 (0, 0) -> (-49.5113, 75.1574)
  line L18 (0, 0) -> (10.8083, 89.3486)
  line L19 (0, 0) -> (-10.8083, 89.3486)
  line L20 (0, 0) -> (-88.3915, -16.9391)
  line L21 (0, 0) -> (-80.8572, 39.5235)
  dimension "d132" = 180
  dimension "d133" = 160
  constraint coincident A0.centre A1.centre
  constraint coincident A13 L12.end
  constraint coincident A1 L12.end
  constraint coincident A13 L13.end
  constraint coincident A13 L14.end
  constraint coincident A13 L15.end
  constraint coincident A13 L16.end
  constraint coincident A0 L17.end
  constraint coincident A13 L18.end
  constraint perpendicular L13 L18
  constraint coincident A13 L19.end
  constraint coincident A13 L20.end
  constraint coincident A13 L21.end
  measures "d132" diameter of A13
  measures "d133" diameter of A14
extrude "Extrude19" cut sketch "Sketch17" against normal blind 10 contours L11 A14 L18 L19 | A0 A13 A14 L17 L21 | A0 A13 A14 L16 L20 | A1 A13 A14 L14 L15 | A1 A13 A14 L12 L13 bodies 1
sketch "Sketch18" plane through (0, 102, 0) normal (0, 1, 0) x (1, 0, 0)
  line L0 (0, 0) -> (-40, 0)
  line L1 (-32.3996, 9.6332) -> (-47.6004, 9.6332)
  line L2 (-47.6004, 9.6332) -> (-47.6004, -9.6332)
  line L3 (-47.6004, -9.6332) -> (-32.3996, -9.6332)
  line L4 (-32.3996, -9.6332) -> (-32.3996, 9.6332)
  line L5 (-32.3996, 9.6332) -> (-47.6004, -9.6332) construction
  line L6 (-47.6004, 9.6332) -> (-32.3996, -9.6332) construction
  point P0 (-40, 0)
  dimension "d136" = 40
  constraint coincident L0.start origin
  constraint horizontal L0
  constraint horizontal L1
  constraint perpendicular L1 L2
  constraint parallel L1 L3
  constraint parallel L2 L4
  constraint coincident L5 P0
  constraint coincident L6 P0
  constraint coincident P0 L0.end
  measures "d136" distance of L0.start P0
extrude "Extrude20" cut sketch "Sketch18" against normal blind 40 bodies 1 2
sketch "Sketch19" plane through (0, 0, -5) normal (0, 0, -1) x (1, 0, 0)
  circle A0 centre (16.5, 41.5) radius 2.9
  circle A1 centre (16.5, 41.5) radius 2
  dimension "d139" = 4
  constraint concentric A0 A1
  measures "d139" diameter of A1
extrude "Extrude21" cut sketch "Sketch19" against normal blind 5 contours A1 bodies 1
sketch "Sketch20" plane through (0, 0, -5) normal (0, 0, -1) x (1, 0, 0)
  circle A0 centre (-40.5, 71.5) radius 2.9
  circle A1 centre (-40.5, 71.5) radius 2
  dimension "d142" = 4
  constraint concentric A0 A1
  measures "d142" diameter of A1
extrude "Extrude22" cut sketch "Sketch20" against normal blind 5 contours A1 bodies 1
